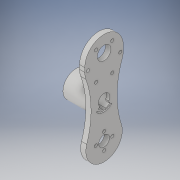
# Autodesk Inventor part: Frame_DC
Saved by Autodesk Inventor 2019 (Build 230136000, 136)
## iProperties
Created: 2019-07-29
Part Number: Frame_DC
Material: Generic
Document SubType Name: Modeling
Designer: 19879326
Density: 1 g/cm^3
Appearance: Default
Author: 19879326
Autodesk Inventor part; units mm, degrees
ref_plane "YZ Plane" through (0, 0, 0) normal (1, 0, 0) x (0, 1, 0)
ref_plane "XZ Plane" through (0, 0, 0) normal (0, 1, 0) x (-1, 0, 0)
ref_plane "XY Plane" through (0, 0, 0) normal (0, 0, 1) x (1, 0, 0)
sketch "Sketch1" plane through (0, 0, 0) normal (1, 0, 0) x (0, 1, 0)
  circle A0 centre (0, 15.5) radius 1.5
  arc A1 (-1.4982, 15.4274) -> (-6.5192, 14.0624) centre (0, 0) ccw
  arc A2 (-7.1664, -13.7438) -> (-1.0845, -15.462) centre (0, 0) ccw
  circle A3 centre (7, 0) radius 6.5
  circle A4 centre (13.4234, 7.75) radius 1.5
  circle A5 centre (13.4234, -7.75) radius 1.5
  circle A6 centre (0, -15.5) radius 1.5
  circle A7 centre (-13.4234, 7.75) radius 1.5
  circle A8 centre (-13.4234, -7.75) radius 1.5
  arc A9 (12.6114, 9.0112) -> (1.4982, 15.4274) centre (0, 0) ccw
  arc A10 (15.4989, 0.1825) -> (14.1097, 6.4162) centre (0, 0) ccw
  arc A11 (12.6114, 9.0112) -> (1.4982, 15.4274) centre (0, 0) ccw
  arc A12 (1.4982, -15.4274) -> (12.6114, -9.0112) centre (0, 0) ccw
  arc A13 (14.1097, -6.4162) -> (14.1097, 6.4162) centre (0, 0) ccw
  arc A14 (-14.1097, 6.4162) -> (-14.1097, -6.4162) centre (0, 0) ccw
  arc A15 (-12.6114, -9.0112) -> (-7.1664, -13.7438) centre (0, 0) ccw
  arc A16 (-6.5192, 14.0624) -> (-12.6114, 9.0112) centre (0, 0) ccw
  arc A17 (-14.1097, 6.4162) -> (-15.4979, 0.2553) centre (0, 0) ccw
  circle A18 centre (-32, 0) radius 5.5
  circle A19 centre (-66.15, 0) radius 5.15
  arc A20 (-60.7004, 16.6299) -> (-60.7004, -16.6299) centre (-66.15, 0) ccw
  circle A21 centre (-58.15, 0) radius 1.5
  circle A22 centre (-66.15, 8) radius 1.5
  circle A23 centre (-74.15, 0) radius 1.5
  circle A24 centre (-66.15, -8) radius 1.5
  arc A25 (-6.2612, -17.4082) -> (-60.7004, -16.6299) centre (-34.6135, -96.2365) ccw
  circle A26 centre (-32, 0) radius 12.5
  arc A27 (-60.7004, 16.6299) -> (-6.2612, 17.4082) centre (-34.6135, 96.2365) ccw
  line L0 (0, 18.5) -> (4, 18.5)
  line L1 (0, -18.5) -> (4, -18.5)
  arc A28 (4, -18.5) -> (4, 18.5) centre (4, 0) ccw
  arc A29 (-6.2612, -17.4082) -> (0, -18.5) centre (0, 0) ccw
  arc A30 (0, 18.5) -> (-6.2612, 17.4082) centre (0, 0) ccw
  point P0 (-33.4158, -12.4731)
  dimension "d4" = 15.5
  dimension "d6" = 13
  dimension "d7" = 7
  dimension "d8" = 3
  dimension "d9" = 15.5
  dimension "d10" = 15.5
  dimension "d11" = 15.5
  dimension "d12" = 15.5
  dimension "d13" = 15.5
  dimension "d14" = 15.5
  dimension "d15" = 39
  dimension "d16" = 34.15
  dimension "d17" = 11
  dimension "d18" = 10.3
  dimension "d19" = 35
  dimension "d20" = 3
  dimension "d22" = 8
  dimension "d23" = 8
  dimension "d24" = 8
  dimension "d25" = 8
  dimension "d84" = 25
  dimension "d85" = 4
  dimension "d86" = 18.5
  dimension "d87" = 18.5
  dimension "d88" = 18.5
  constraints: 47 point on circle, 30 centre point, 9 tangent, 7 concentric, 7 vertical alignment, 6 equal radius, 6 horizontal alignment, 5 coincident, 4 end point, 2 horizontal, 5 other
  measures "d4" radius of A1
  measures "d6" diameter of A3
  measures "d7" distance of point (0, 0) A3.centre
  measures "d8" diameter of A0
  measures "d9" distance of A0.centre A4.centre
  measures "d10" distance of A4.centre A5.centre
  measures "d11" distance of point (0, -15.5) A5.centre
  measures "d12" distance of A8.centre point (0, -15.5)
  measures "d13" distance of A7.centre A8.centre
  measures "d14" distance of A7.centre A0.centre
  measures "d15" distance of A3.centre A18.centre
  measures "d16" distance of A19.centre A18.centre
  measures "d17" diameter of A18
  measures "d18" diameter of A19
  measures "d19" diameter of A20
  measures "d20" diameter of A21
  measures "d22" distance of A19.centre A21.centre
  measures "d23" distance of A23.centre A19.centre
  measures "d24" distance of A22.centre A19.centre
  measures "d25" distance of A24.centre A19.centre
  measures "d84" diameter of A26
  measures "d85" distance of L0.end L0.start
  measures "d86" radius of A30
  measures "d87" radius of A29
  measures "d88" radius of A28
extrude "Extrusion1" add sketch "Sketch1" along normal blind 5 contours A0 A9 A4 A10 A13 A5 A12 A6 A2 A15 A8 A14 A7 A16 A1 | A27 A26 A25 A20 | A27 A30 L0 A28 L1 A29 A25 A26 | A26
sketch "Sketch3" plane through (0, 0, 0) normal (-1, 0, 0) x (0, 0, 1)
  circle A0 centre (0, -32) radius 7.6
  circle A1 centre (0, -32) radius 5.5 projected
  point P0 (0, 0)
  dimension "d31" = 15.2
  constraints: 1 centre point, 1 concentric
  measures "d31" diameter of A0
extrude "Extrusion2" cut sketch "Sketch3" against normal blind 2
sketch "Sketch4" plane through (0, 0, 0) normal (-1, 0, 0) x (0, 0, 1)
  arc A0 (-11.4564, -37) -> (-11.4564, -27) centre (0, -32) ccw
  circle A1 centre (0, -32) radius 7.6 projected
  line L0 (-20, -49.15) -> (-20, 0) projected
  line L1 (-20, -40) -> (-20, -24)
  circle A2 centre (0, -32) radius 12.5
  point P0 (0, 0)
  point P1 (-18.5, 0)
  point P2 (-20, -32)
  dimension "d34" = 25
  constraints: 2 centre point, 2 concentric, 2 end point, 2 point on circle, 1 coincident, 1 horizontal alignment, 1 midpoint, 2 other
  measures "d34" diameter of A0
extrude "Extrusion3" add sketch "Sketch4" along normal blind 22
sketch "Sketch6" plane through (-22, 0, 0) normal (-1, 0, 0) x (0, 0, 1)
  arc A0 (-1.3197, -39.4845) -> (1.3197, -39.4845) centre (0, -32) ccw
  circle A1 centre (0, -32) radius 7.6 projected
  arc A2 (-1.5802, -40.9618) -> (-1.3197, -39.4845) centre (-1.45, -40.2231) ccw
  arc A3 (1.3197, -39.4845) -> (1.5802, -40.9618) centre (1.45, -40.2231) ccw
  line L0 (0, -32) -> (0, -39.6)
  circle A4 centre (0, -32) radius 7.6 projected
  arc A5 (1.5802, -40.9618) -> (-1.5802, -40.9618) centre (0, -32) ccw
  arc A6 (-7.1418, -39.1418) -> (7.1418, -39.1418) centre (0, -32) ccw
  arc A7 (-6.4347, -38.4347) -> (-7.1418, -39.1418) centre (-6.7882, -38.7882) ccw
  arc A8 (7.1418, -39.1418) -> (6.4347, -38.4347) centre (6.7882, -38.7882) ccw
  point P0 (0, 0)
  dimension "d48" = 10
  dimension "d49" = 10
  dimension "d50" = 45
  dimension "d51" = 45
  dimension "d52" = 1.5
  dimension "d53" = 1
  constraints: 19 point on circle, 7 centre point, 7 tangent, 2 coincident, 2 concentric, 2 end point, 2 equal radius, 1 vertical
  measures "d52" diameter of A2
  measures "d53" diameter of A7
extrude "Extrusion5" cut sketch "Sketch6" against normal blind 28 contours A0 A3 A5 A8 A6 A7 A2
sketch "Sketch7" plane through (5, 0, 0) normal (1, 0, 0) x (0, 0, -1)
  arc A0 (-5.374, -37.374) -> (5.374, -37.374) centre (0, -32) ccw
  arc A1 (1.3197, -39.4845) -> (-1.3197, -39.4845) centre (0, -32) ccw projected
  arc A2 (-1.3197, -39.4845) -> (1.3197, -39.4845) centre (0, -32) ccw projected
  arc A3 (-5.0445, -36.521) -> (-5.374, -37.374) centre (-5.0205, -37.0205) ccw
  arc A4 (5.374, -37.374) -> (5.0445, -36.521) centre (5.0205, -37.0205) ccw
  arc A5 (7.1418, -39.1418) -> (6.4347, -38.4347) centre (6.7882, -38.7882) ccw projected
  arc A6 (-6.4347, -38.4347) -> (-7.1418, -39.1418) centre (-6.7882, -38.7882) ccw projected
  line L0 (0, -32) -> (0, -39.6)
  arc A7 (-1.3197, -39.4845) -> (1.3197, -39.4845) centre (0, -32) ccw projected
  arc A8 (-5.0445, -36.521) -> (-4.4375, -35.2493) centre (-5.083, -35.722) ccw
  arc A9 (4.4375, -35.2493) -> (5.0445, -36.521) centre (5.083, -35.722) ccw
  circle A10 centre (0, -32) radius 5.5 projected
  arc A11 (-4.4375, -35.2493) -> (4.4375, -35.2493) centre (0, -32) ccw
  point P0 (0, 0)
  dimension "d56" = 45
  dimension "d57" = 45
  dimension "d61" = 0.8
  constraints: 18 point on circle, 7 tangent, 6 centre point, 4 equal radius, 2 end point, 1 coincident, 1 concentric
  measures "d61" radius of A8
extrude "Extrusion6" cut sketch "Sketch7" against normal blind 5 contours A3 A8 A10 L0 A0 | A0 L0 A10 A9 A4
body "Solid1"
